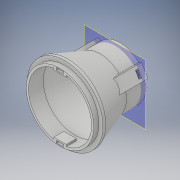
# Autodesk Inventor part: endkappen_V2
Saved by Autodesk Inventor 2017 (Build 210142000, 142)
## iProperties
Part Number: endkappen_V2
Material: Generisch
Document SubType Name: Modeling
Designer: Fabio
Density: 1 g/cm^3
Appearance: Vorgabe
Author: Fabio
Autodesk Inventor part; units mm, degrees
ref_plane "YZ Plane" through (0, 0, 0) normal (1, 0, 0) x (0, 1, 0)
ref_plane "XZ Plane" through (0, 0, 0) normal (0, 1, 0) x (-1, 0, 0)
ref_plane "XY Plane" through (0, 0, 0) normal (0, 0, 1) x (1, 0, 0)
sketch "Skizze2" plane through (0, 0, 0) normal (1, 0, 0) x (0, 1, 0)
  line L0 (40.2024, 14.6469) -> (11.7576, 25)
  line L1 (0, 0) -> (48.6481, 0)
  line L2 (47.4748, 14.5263) -> (47.4748, 20.6434)
  line L3 (47.4748, 20.6434) -> (31.9696, 20.6434)
  line L4 (6.2626, 30) -> (31.9696, 20.6434)
  line L5 (4, 30) -> (4, 26.75)
  line L6 (4, 26.75) -> (0, 26.75)
  line L7 (6.2626, 30) -> (4, 30)
  line L8 (11.7576, 25) -> (0, 25)
  line L9 (0, 25) -> (0, 26.75)
  line L10 (0, 0) -> (0, 25) construction
  line L11 (47.4748, 14.5263) -> (40.8864, 14.5263)
  arc A0 (40.2024, 14.6469) -> (40.8864, 14.5263) centre (40.8864, 16.5263) ccw
  point P0 (40.5337, 14.5263)
  dimension "d22" = 20
  dimension "d115" = 15.5052
  dimension "d164" = 60
  dimension "d166" = 53.5
  dimension "d167" = 50
  dimension "d168" = 4
  dimension "d169" = 3.25
  dimension "d171" = 47.4748
  dimension "d172" = 29.0527
  dimension "d173" = 41.2869
  dimension "d174" = 40.5337
  dimension "d175" = 2
  constraints: 24 end point, 5 horizontal, 2 point on circle, 2 point on line, 2 tangent, 2 vertical, 1 centre point, 1 parallel, 1 perpendicular
  measures "d22" angle of L1 L0
  measures "d115" distance of L2.end L3.end
  measures "d164" diameter of L7 L1
  measures "d166" diameter of L6 L1
  measures "d167" diameter of L8 L1
  measures "d168" distance of L5.end L6.end
  measures "d169" distance of L5.start L5.end
  measures "d171" horizontal distance of L8.end L2.end
  measures "d172" diameter of L11 L1
  measures "d173" diameter of L3 L1
  measures "d174" distance from line of L10 point (40.534, 14.526)
  measures "d175" radius of A0
revolve "Umdrehung1" add sketch "Skizze2" angle 360 about axis through (0, 0, 0) along (0, 1, 0)
sketch "Skizze15" plane through (0, 47.4748, 0) normal (0, 1, 0) x (1, 0, 0)
  circle A0 centre (0, 0) radius 20.6434 projected
  circle A1 centre (0, 0) radius 14.5263 projected
  line L0 (-5, 18.6434) -> (-5, 22.6434)
  line L1 (-5, 22.6434) -> (5, 22.6434)
  line L2 (5, 22.6434) -> (5, 18.6434)
  line L3 (5, 18.6434) -> (-5, 18.6434)
  line L4 (-5, 18.6434) -> (5, 22.6434) construction
  line L5 (-5, 22.6434) -> (5, 18.6434) construction
  line L6 (-17.1098, -15.6518) -> (-22.1098, -6.9916)
  line L7 (-22.1098, -6.9916) -> (-18.6457, -4.9916)
  line L8 (-18.6457, -4.9916) -> (-13.6457, -13.6518)
  line L9 (-13.6457, -13.6518) -> (-17.1098, -15.6518)
  line L10 (22.1098, -6.9916) -> (17.1098, -15.6518)
  line L11 (17.1098, -15.6518) -> (13.6457, -13.6518)
  line L12 (13.6457, -13.6518) -> (18.6457, -4.9916)
  line L13 (18.6457, -4.9916) -> (22.1098, -6.9916)
  point P0 (0, 20.6434)
  dimension "d129" = 10
  dimension "d130" = 4
  dimension "d131" = 18.6434
  dimension "d134" = 360
  constraints: 28 end point, 2 midpoint, 2 parallel, 1 perpendicular, 1 vertical, 1 vertical alignment, 26 other
  measures "d129" distance of L0.end L1.end
  measures "d130" distance of L1.end L2.end
  measures "d131" distance from line of point (0, 0) L3
extrude "Extrusion12" add sketch "Skizze15" against normal blind 25 contours L2 L3 L0 A0 | A0 L0 L1 L2 | L13 L10 L11 A0 | A0 L11 L12 L13 | L7 L8 L9 A0 | A0 L9 L6 L7
delete faces "Fläche löschen5" heal yes whole lump no faces at (0, 24.7239, -18.6434) (-0.5603, 22.4748, -19.4397)
delete faces "Fläche löschen6" heal yes whole lump no faces at (17.1154, 22.4748, 9.2346) (16.1457, 24.7239, 9.3217)
delete faces "Fläche löschen7" heal yes whole lump no faces at (-16.5551, 22.4748, 10.2051) (-16.1457, 24.7239, 9.3217)
ref_plane "Arbeitsebene2" through (-5, 43.4748, -22.6434) normal (0, 1, 0) x (1, 0, 0)
sketch "Skizze16" plane through (-5, 43.4748, -22.6434) normal (0, 1, 0) x (1, 0, 0)
  line L0 (-17.1098, -29.635) -> (-12.1098, -38.2953) projected
  line L1 (0, 0) -> (10, 0) projected
  line L2 (2.15, 5.7) -> (7.85, 5.7)
  line L3 (7.85, 5.7) -> (7.85, -5.7)
  line L4 (7.85, -5.7) -> (2.15, -5.7)
  line L5 (2.15, -5.7) -> (2.15, 5.7)
  line L6 (2.15, 5.7) -> (7.85, -5.7) construction
  line L7 (7.85, 5.7) -> (2.15, -5.7) construction
  line L8 (-20.9711, -34.347) -> (-11.0984, -28.647)
  line L9 (-18.1211, -39.2833) -> (-20.9711, -34.347)
  line L10 (-8.2484, -33.5833) -> (-18.1211, -39.2833)
  line L11 (-11.0984, -28.647) -> (-8.2484, -33.5833)
  line L12 (28.1211, -39.2833) -> (18.2484, -33.5833)
  line L13 (30.9711, -34.347) -> (28.1211, -39.2833)
  line L14 (21.0984, -28.647) -> (30.9711, -34.347)
  line L15 (18.2484, -33.5833) -> (21.0984, -28.647)
  point P0 (5, -22.6434)
  point P1 (5, 0)
  dimension "d139" = 5.7
  dimension "d140" = 11.4
  dimension "d143" = 360
  constraints: 28 end point, 3 midpoint, 2 parallel, 1 horizontal, 1 perpendicular, 25 other
  measures "d139" distance of L3.end L4.end
  measures "d140" distance of L2.end L3.end
extrude "Extrusion13" cut sketch "Skizze16" against normal blind 2
sketch "Skizze17" plane through (-5, 47.4748, -22.6434) normal (0, 1, 0) x (1, 0, 0)
  line L0 (0, 0) -> (10, 0) projected
  line L1 (5, -22.6434) -> (5, -2.85) construction
  point P0 (-12.1416, -32.5402)
  point P1 (22.1416, -32.5402)
  dimension "d147" = 2.85
  dimension "d150" = 360
  constraints: 2 end point, 1 coincident, 1 vertical, 4 other
  measures "d147" distance from line of L0 L1.end
hole "Bohrung3" at (0, 47.4748, -19.7934) at (-17.1416, 47.4748, 9.8967) at (17.1416, 47.4748, 9.8967) direction (0, -1, 0) diameter 3.3 depth 15 tip angle 118
sketch "Skizze18" plane through (0, 0, 0) normal (0, -1, 0) x (1, 0, 0)
  circle A0 centre (0, 0) radius 25 projected
  line L0 (5, -23) -> (-5, -23)
  line L1 (-5, -23) -> (-5, -25)
  line L2 (-5, -25) -> (5, -25)
  line L3 (5, -25) -> (5, -23)
  line L4 (5, -23) -> (-5, -25) construction
  line L5 (-5, -23) -> (5, -25) construction
  line L6 (0, -24) -> (0, 0) construction
  line L7 (0, 0) -> (9.0804, 0) construction
  line L8 (5, 23) -> (-5, 23)
  line L9 (-5, 23) -> (-5, 25)
  line L10 (-5, 25) -> (5, 25)
  line L11 (5, 25) -> (5, 23)
  dimension "d176" = 10
  dimension "d177" = 2
  dimension "d178" = 23
  constraints: 24 end point, 4 symmetric about line, 2 horizontal, 2 midpoint, 2 parallel, 1 perpendicular, 1 vertical
  measures "d176" distance of L2.end L1.end
  measures "d177" distance of L0.end L1.end
  measures "d178" distance from line of point (0, 0) L0
extrude "Extrusion14" add sketch "Skizze18" against normal blind 8 contours L11 L8 L9 A0 | A0 L10 L11 | L3 L2 A0 | A0 L1 L0 L3 | A0 L9 L10 | L2 L1 A0
sketch "Skizze19" plane through (0, 0, 0) normal (0, -1, 0) x (1, 0, 0)
  line L0 (-2.85, -24) -> (2.85, -24)
  line L1 (2.85, -24) -> (2.85, -26)
  line L2 (2.85, -26) -> (-2.85, -26)
  line L3 (-2.85, -26) -> (-2.85, -24)
  arc A0 (-5, -24.4949) -> (5, -24.4949) centre (0, 0) ccw projected
  line L4 (-2.85, -24) -> (2.85, -26) construction
  line L5 (2.85, -24) -> (-2.85, -26) construction
  line L6 (0, -25) -> (0, 0) construction
  line L7 (0, 0) -> (9.7237, 0) construction
  line L8 (-2.85, 24) -> (2.85, 24)
  line L9 (2.85, 24) -> (2.85, 26)
  line L10 (2.85, 26) -> (-2.85, 26)
  line L11 (-2.85, 26) -> (-2.85, 24)
  dimension "d181" = 5.7
  dimension "d182" = 2
  constraints: 24 end point, 4 symmetric about line, 2 horizontal, 2 midpoint, 2 parallel, 1 perpendicular, 1 point on circle, 1 vertical
  measures "d181" distance of L1.end L2.end
  measures "d182" distance of L0.end L1.end
extrude "Extrusion15" cut sketch "Skizze19" against normal blind 5.7
